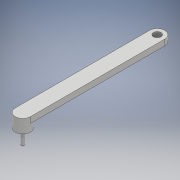
# Autodesk Inventor part: Arm - stabilizer linkage
Saved by Autodesk Inventor 2017 (Build 210142000, 142)
## iProperties
Created: 2016-05-05
Part Number: Arm - stabilizer linkage
Material: Generic
Document SubType Name: Modeling
Designer: alist
Density: 1 g/cm^3
Appearance: Default
Author: alist
## iProperties of the stored document Arm - stabilizer linkage_3DPrint.ipt
Created: 2017-01-15
Part Number: Arm - stabilizer linkage_3DPrint
Material: Generic
Document SubType Name: Modeling
Designer: Alistair
Density: 1 g/cm^3
Appearance: Default
Author: Alistair
Autodesk Inventor part; units mm, degrees
ref_plane "YZ Plane" through (0, 0, 0) normal (1, 0, 0) x (0, 1, 0)
ref_plane "XZ Plane" through (0, 0, 0) normal (0, 1, 0) x (-1, 0, 0)
sketch "Sketch1" plane through (0, 0, 0) normal (0, 0, 1) x (1, 0, 0)
  circle A0 centre (-24.3, 72.0995) radius 4.5 projected
  circle A1 centre (-24.3, 72.0995) radius 9
  circle A2 centre (-24.3, 232.0995) radius 9
  line L0 (-33.3, 72.0995) -> (-33.3, 232.0995)
  line L1 (-15.3, 72.0995) -> (-15.3, 232.0995)
  point P0 (0, 0)
  dimension "d0" = 4.5
  dimension "d1" = 160
  dimension "d2" = 18
  constraints: 4 end point, 4 point on circle, 2 centre point, 2 vertical, 1 coincident
  measures "d0" radial gap between concentric circles of A0 A1
  measures "d1" distance of A0.centre point (-24.3, 232.099)
  measures "d2" diameter of A2
extrude "Extrusion1" add sketch "Sketch1" along normal blind 7 contours A0 | A1 | A1 L0 A2 L1 | A2
sketch "Sketch2" plane through (0, 0, 0) normal (0, 0, -1) x (-1, 0, 0)
  arc A0 (15.3, 72.0995) -> (33.3, 72.0995) centre (24.3, 72.0995) ccw projected
  circle A1 centre (24.3, 72.0995) radius 9
  point P0 (0, 0)
  constraints: 1 coincident, 1 horizontal alignment, 2 other
extrude "Extrusion2" add sketch "Sketch2" along normal blind 9
hole "Hole1" at (-24.3, 232.0995, 7) direction (0, 0, -1) diameter 9 end through all
sketch "Sketch3" plane through (-24.3, 72.0995, -9) normal (0, 0, -1) x (-1, 0, 0)
  circle A0 centre (0, 0) radius 3
  point P0 (-24.3, -72.0995)
  dimension "d26" = 6
  constraints: 1 centre point
  measures "d26" diameter of A0
extrude "Extrusion3" add sketch "Sketch3" along normal blind 1
sketch "Sketch4" plane through (-24.3, 72.0995, -10) normal (0, 0, -1) x (-1, 0, 0)
  circle A0 centre (0, 0) radius 1.95
  point P0 (-24.3, -72.0995)
  dimension "d29" = 3.9
  constraints: 1 centre point
  measures "d29" diameter of A0
ref_plane "Work Plane1" through (-48.2164, 25.8529, -27) normal (0, 0, -1) x (0.4885851, 0.8725162, 0)
extrude "Extrusion4" add sketch "Sketch4" along normal up to surface (17 mm away)
sketch "Sketch5" plane through (0, 0, 0) normal (0, 0, -1) x (-1, 0, 0)
  circle A0 centre (24.3, 232.0995) radius 4.5 projected
  circle A1 centre (24.3, 232.0995) radius 3
  point P0 (0, 0)
  dimension "d32" = 6
  constraints: 1 centre point, 1 coincident
  measures "d32" diameter of A1
extrude "Extrusion5" add sketch "Sketch5" against normal blind 1
chamfer "Chamfer1" distance 1.5 angle 45 1 edges at (-24.3, 236.5995, 1)
chamfer "Chamfer2" distance 0.8 angle 45 1 edges at (-22.35, 72.0995, -27)
body "Solid1"
